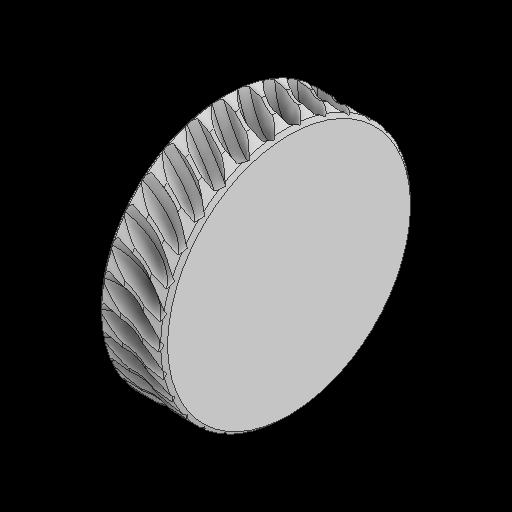
# Autodesk Inventor part: Corona
Saved by Autodesk Inventor 2027 (Build 310192000, 192)
## iProperties
Created: 2026-05-13
Part Number: Corona
Material: Genérico
Document SubType Name: Modeling
Designer: giova
Density: 1 g/cm^3
Appearance: Valor por defecto
Author: giova
Autodesk Inventor part; units mm, degrees
ref_plane "YZ Plane" through (0, 0, 0) normal (1, 0, 0) x (0, 1, 0)
ref_plane "XZ Plane" through (0, 0, 0) normal (0, 1, 0) x (-1, 0, 0)
ref_plane "Plano de trabajo1" through (0, 0, 0) normal (0.8660254, 0, 0.5) x (0, 1, 0)
sketch "Boceto1" plane through (0, 0, 0) normal (0, 0, 1) x (1, 0, 0)
  line L0 (21.9125, 39.0673) -> (21.9125, -41.3115)
  line L1 (21.9125, -41.3115) -> (-21.9125, -41.3115)
  line L2 (-21.9125, -41.3115) -> (-21.9125, 39.0673)
  arc A0 (-7.1232, 41.3115) -> (7.1232, 41.3115) centre (0, 60) ccw
  line L3 (-19.5632, 41.3115) -> (-21.9125, 39.0673)
  line L4 (0, 60) -> (0, 51.4857) construction
  line L5 (19.5632, 41.3115) -> (21.9125, 39.0673)
  line L6 (-19.5632, 41.3115) -> (-7.1232, 41.3115)
  line L7 (7.1232, 41.3115) -> (19.5632, 41.3115)
  point P0 (0, 0)
  point P1 (0, 41.3115)
  point P2 (21.9125, 0)
  dimension "d1" = 43.825
  dimension "d3" = 40
  dimension "d4" = 60
  dimension "d5" = 46.31
  constraints: 16 end point, 3 parallel, 2 horizontal, 2 perpendicular, 2 point on circle, 2 symmetric about line, 2 vertical alignment, 1 centre point, 1 horizontal alignment, 1 point on line, 1 vertical
  measures "d1" distance between parallel lines of L0 L2
  measures "d3" diameter of A0
  measures "d4" distance of point (0, 0) L4.start
  measures "d5" angle of L3 L4
revolve "Revolución1" add sketch "Boceto1" angle 360 about axis through (21.9125, -41.3115, 0) along (-1, 0, 0)
sketch "Boceto2" plane through (21.9125, -41.3115, 0) normal (1, 0, 0) x (0, 0, -1)
  circle A0 centre (0, 0) radius 75
  point P0 (0, 41.3115)
  dimension "d7" = 150
  constraints: 1 centre point
  measures "d7" diameter of A0
surface extrude "SuperficieExtrusión1" sketch "Boceto2" against normal blind 43.835 shown no curves A0
sketch "Boceto3" plane through (0, 0, 0) normal (0.8660254, 0, 0.5) x (0, 1, 0)
  line L0 (60, 6.8358) -> (60, -6.8358)
  line L1 (60, -6.8358) -> (40.835, -6.8358)
  line L2 (40.835, -6.8358) -> (30, -2.8921)
  line L3 (30, -2.8921) -> (30, 2.8921)
  line L4 (30, 2.8921) -> (40.835, 6.8358)
  line L5 (40.835, 6.8358) -> (60, 6.8358)
  line L6 (35, 0) -> (35, -4.712) construction
  point P0 (0, 0)
  point P1 (60, 0)
  point P2 (60, 0)
  point P3 (30, 0)
  dimension "d10" = 60
  dimension "d11" = 30
  dimension "d12" = 20
  dimension "d13" = 20
  dimension "d14" = 19.165
  dimension "d15" = 25
  dimension "d16" = 4.712
  constraints: 14 end point, 3 horizontal alignment, 2 midpoint, 2 parallel, 2 vertical, 1 coincident, 1 perpendicular, 1 point on line
  measures "d10" distance of point (0, 0) point (60, 0)
  measures "d11" distance between parallel lines of L3 L0
  measures "d12" angle of L2 L1
  measures "d13" angle of L4 L5
  measures "d14" distance of L0.end L1.end
  measures "d15" distance from line of L6.start L0
  measures "d16" distance of L6.start L6.end
revolve "Revolución2" cut sketch "Boceto3" angle 360 about axis through (-3.4179, 60, 5.9199) along (0.5, 0, -0.8660254)
pattern_circular "Patrón circular1" count 30 over 360 about axis through (20.7379, -41.3115, 0) along (-1, 0, 0) of "Revolución2"
